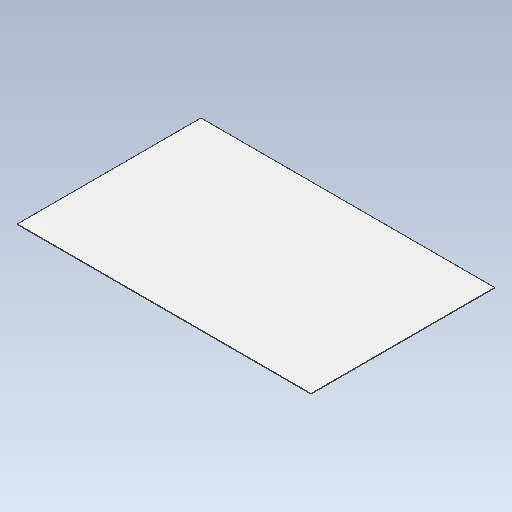
# Autodesk Inventor part: panel
Saved by Autodesk Inventor 2020 (Build 240168000, 168)
## iProperties
Created: 2020-06-26
Part Number: panel
Material: Generic
Document SubType Name: Modeling
Designer: Abbas
Density: 1 g/cm^3
Appearance: Default
Author: Abbas
Autodesk Inventor part; units mm, degrees
ref_plane "YZ Plane" through (0, 0, 0) normal (1, 0, 0) x (0, 1, 0)
ref_plane "XZ Plane" through (0, 0, 0) normal (0, 1, 0) x (-1, 0, 0)
ref_plane "XY Plane" through (0, 0, 0) normal (0, 0, 1) x (1, 0, 0)
sketch "Sketch1" plane through (0, 0, 0) normal (0, 1, 0) x (-1, 0, 0)
  line L0 (513, 317) -> (-513, 317)
  line L1 (-513, 317) -> (-513, -317)
  line L2 (-513, -317) -> (513, -317)
  line L3 (513, -317) -> (513, 317)
  line L4 (513, 317) -> (-513, -317) construction
  line L5 (-513, 317) -> (513, -317) construction
  line L6 (523, 327) -> (-523, 327)
  line L7 (-523, 327) -> (-523, -327)
  line L8 (-523, -327) -> (523, -327)
  line L9 (523, -327) -> (523, 327)
  line L10 (523, 327) -> (-523, -327) construction
  line L11 (-523, 327) -> (523, -327) construction
  point P0 (0, 0)
  dimension "d0" = 1026
  dimension "d1" = 634
  dimension "d2" = 1046
  dimension "d3" = 654
  constraints: 24 end point, 4 midpoint, 4 parallel, 2 horizontal, 2 perpendicular
  measures "d0" distance of L2.end L1.end
  measures "d1" distance of L1.end L0.end
  measures "d2" distance of L8.end L7.end
  measures "d3" distance of L7.end L6.end
extrude "Extrusion1" add sketch "Sketch1" along normal blind 2
extrude "Extrusion2" add sketch "Sketch1" along normal blind 2 contours L3 L2 L1 L0
body "Solid1"
